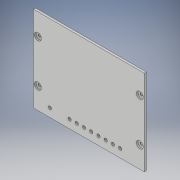
# Autodesk Inventor part: Ra-Manager_Painel-Placas_Relays
Saved by Autodesk Inventor 2019.4 (Build 234330000, 330)
## iProperties
Created: 2020-03-19
Part Number: Ra-Manager_Painel-Placas_Relays
Material: Aço, carbono
Document SubType Name: Modeling
Designer: caio.santos
Density: 7.85 g/cm^3
Appearance: Padrão
Author: caio.santos
Autodesk Inventor part; units mm, degrees
ref_plane "YZ Plane" through (0, 0, 0) normal (1, 0, 0) x (0, 1, 0)
ref_plane "XZ Plane" through (0, 0, 0) normal (0, 1, 0) x (-1, 0, 0)
ref_plane "XY Plane" through (0, 0, 0) normal (0, 0, 1) x (1, 0, 0)
sketch "Esboço1" plane through (0, 0, 0) normal (0, 0, 1) x (1, 0, 0)
  line L0 (-50.5, -39) -> (50.5, -39)
  line L1 (50.5, -39) -> (50.5, 39)
  line L2 (50.5, 39) -> (-50.5, 39)
  line L3 (-50.5, 39) -> (-50.5, -39)
  point P0 (0, 0)
  dimension "d2" = 101
  dimension "d3" = 78
  dimension "d4" = 101
  dimension "d5" = 50.5
  dimension "d6" = 39
  constraints: 8 end point, 1 parallel, 1 perpendicular, 1 vertical
  measures "d2" distance of L0.start L0.end
  measures "d3" distance of L0.end L1.end
  measures "d4" distance of L1.end L2.end
  measures "d5" distance from line of point (0, 0) L1
  measures "d6" distance from line of point (0, 0) L2
extrude "Extrusão1" add sketch "Esboço1" against normal blind 2
sketch "Esboço2" plane through (0, 0, 0) normal (0, 0, 1) x (1, 0, 0)
  line L0 (-50.5, -39) -> (-50.5, 39) projected
  line L1 (-42.5, -39) -> (-42.5, 39) construction
  line L2 (42.5, -39) -> (42.5, 39) construction
  line L3 (-46.5, 39) -> (-46.5, -39) construction
  line L4 (-50.5, 39) -> (50.5, 39) projected
  line L5 (46.5, 39) -> (46.5, -39) construction
  line L6 (50.5, 39) -> (50.5, -39) projected
  line L7 (-50.5, -19.5) -> (50.5, -19.5) construction
  line L8 (-50.5, 19.5) -> (50.5, 19.5) construction
  point P0 (0, 0)
  point P1 (-46.5, 19.5)
  point P2 (-46.5, -19.5)
  point P3 (46.5, -19.5)
  point P4 (46.5, 19.5)
  constraints: 13 point on line, 12 end point, 2 perpendicular, 1 parallel
hole "Furo1" at (-46.5, 19.5, 0) at (-46.5, -19.5, 0) at (46.5, -19.5, 0) at (46.5, 19.5, 0) direction (0, 0, -1) diameter 2.459 end through all counterbore diameter 6.5 counterbore depth 1.5 thread size "M3x0.5" class "6H" standard "ANSI Metric M Profile"
sketch "Esboço3" plane through (0, 0, -2) normal (0, 0, -1) x (-1, 0, 0)
  line L0 (39.7375, -31.6586) -> (-39.7375, -31.6586) projected
  line L1 (-29.1874, -30.9886) -> (-27.9874, -30.9886) projected
  line L2 (-27.9874, -30.9886) -> (-27.9374, -31.5336) projected
  line L3 (-29.1874, -30.9886) -> (-29.2374, -31.5336) projected
  line L4 (-22.5874, -30.9886) -> (-21.3874, -30.9886) projected
  line L5 (-22.5874, -30.9886) -> (-22.6374, -31.5336) projected
  line L6 (-21.3874, -30.9886) -> (-21.3374, -31.5336) projected
  line L7 (-21.3874, -30.9886) -> (-21.3874, -30.9886) projected
  line L8 (-15.9874, -30.9886) -> (-14.7874, -30.9886) projected
  line L9 (-15.9874, -30.9886) -> (-16.0374, -31.5336) projected
  line L10 (-14.7874, -30.9886) -> (-14.7374, -31.5336) projected
  line L11 (-9.3874, -30.9886) -> (-8.1874, -30.9886) projected
  line L12 (-8.1874, -30.9886) -> (-8.1374, -31.5336) projected
  line L13 (-9.3874, -30.9886) -> (-9.4374, -31.5336) projected
  line L14 (-2.7874, -30.9886) -> (-1.5874, -30.9886) projected
  line L15 (-2.7874, -30.9886) -> (-2.8374, -31.5336) projected
  line L16 (-1.5874, -30.9886) -> (-1.5374, -31.5336) projected
  line L17 (3.8127, -30.9886) -> (5.0127, -30.9886) projected
  line L18 (5.0127, -30.9886) -> (5.0627, -31.5336) projected
  line L19 (3.8127, -30.9886) -> (3.7627, -31.5336) projected
  line L20 (10.4126, -30.9886) -> (11.6126, -30.9886) projected
  line L21 (10.4126, -30.9886) -> (10.4126, -30.9886) projected
  line L22 (10.4126, -30.9886) -> (10.3626, -31.5336) projected
  line L23 (11.6126, -30.9886) -> (11.6626, -31.5336) projected
  line L24 (17.0126, -30.9886) -> (18.2126, -30.9886) projected
  line L25 (17.0126, -30.9886) -> (16.9626, -31.5336) projected
  line L26 (18.2126, -30.9886) -> (18.2626, -31.5336) projected
  line L27 (35.0474, -31.0186) -> (35.9774, -31.0186) projected
  line L28 (36.3874, -31.6586) -> (36.3874, -31.0186) projected
  line L29 (34.6374, -31.6586) -> (34.6374, -31.0186) projected
  line L30 (35.0474, -31.0186) -> (34.6374, -31.0186) projected
  line L31 (36.3874, -31.0186) -> (35.9774, -31.0186) projected
  line L32 (-28.5874, -31.3386) -> (36.3874, -31.3386) construction
  circle A0 centre (35.5124, -31.3386) radius 1.5
  circle A1 centre (-28.5874, -31.3386) radius 1.5
  circle A2 centre (17.6126, -31.3386) radius 1.5
  circle A3 centre (11.0126, -31.3386) radius 1.5
  circle A4 centre (4.4127, -31.3386) radius 1.5
  circle A5 centre (-2.1874, -31.3386) radius 1.5
  circle A6 centre (-8.7874, -31.3386) radius 1.5
  circle A7 centre (-15.3874, -31.3386) radius 1.5
  circle A8 centre (-21.9874, -31.3386) radius 1.5
  point P0 (0, 0)
  dimension "d23" = 3
  dimension "d24" = 3
  dimension "d25" = 3
  dimension "d26" = 3
  dimension "d27" = 3
  dimension "d28" = 3
  dimension "d29" = 3
  dimension "d30" = 3
  dimension "d31" = 3
  dimension "d32" = 0.32
  dimension "d33" = 0.875
  dimension "d34" = 18.7748
  dimension "d35" = 25.3748
  dimension "d36" = 31.9748
  dimension "d37" = 38.5748
  dimension "d38" = 45.1748
  dimension "d39" = 51.7748
  dimension "d40" = 58.3748
  dimension "d41" = 64.9748
  constraints: 9 centre point, 1 coincident, 1 horizontal, 1 midpoint, 10 other
  measures "d23" diameter of A0
  measures "d24" diameter of A1
  measures "d25" diameter of A2
  measures "d26" diameter of A3
  measures "d27" diameter of A4
  measures "d28" diameter of A5
  measures "d29" diameter of A6
  measures "d30" diameter of A7
  measures "d31" diameter of A8
  measures "d32" distance from line of A0.centre L0
  measures "d33" distance from line of A0.centre L28
  measures "d34" distance from line of A2.centre L28
  measures "d35" distance from line of A3.centre L28
  measures "d36" distance from line of A4.centre L28
  measures "d37" distance from line of A5.centre L28
  measures "d38" distance from line of A6.centre L28
  measures "d39" distance from line of A7.centre L28
  measures "d40" distance from line of A8.centre L28
  measures "d41" distance from line of point (-28.587, -31.339) L28
extrude "Extrusão2" cut sketch "Esboço3" against normal blind 10
